Autodesk Fusion 360 part; units mm, degrees
(part 3 of 4)
  line L277 (275.3106, 39.6541) -> (275.3106, 39.9415)
  line L278 (275.3106, 39.9415) -> (276.614, 39.9415)
  arc A250 (276.614, 39.9415) -> (277.114, 40.4415) centre (276.614, 40.4415) ccw
  line L279 (277.114, 40.4415) -> (277.114, 40.6099)
  arc A251 (277.614, 41.1099) -> (277.114, 40.6099) centre (277.614, 40.6099) ccw
  line L280 (277.614, 41.1099) -> (279.662, 41.1099)
  arc A252 (280.162, 40.6099) -> (279.662, 41.1099) centre (279.662, 40.6099) ccw
  line L281 (280.162, 40.6099) -> (280.162, 40.4415)
  arc A253 (280.162, 40.4415) -> (280.662, 39.9415) centre (280.662, 40.4415) ccw
  line L282 (280.662, 39.9415) -> (281.4654, 39.9415)
  arc A254 (281.9654, 39.4415) -> (281.4654, 39.9415) centre (281.4654, 39.4415) ccw
  line L283 (281.9654, 39.4415) -> (281.9654, 34.3455)
  arc A255 (281.9654, 34.3455) -> (282.4654, 33.8455) centre (282.4654, 34.3455) ccw
  arc A256 (212.075, 26.8375) -> (212.575, 26.3375) centre (212.575, 26.8375) ccw
  line L284 (212.075, 26.8375) -> (212.075, 39.8375)
  arc A257 (212.575, 40.3375) -> (212.075, 39.8375) centre (212.575, 39.8375) ccw
  line L285 (212.575, 40.3375) -> (225.575, 40.3375)
  arc A258 (226.075, 39.8375) -> (225.575, 40.3375) centre (225.575, 39.8375) ccw
  line L286 (226.075, 39.8375) -> (226.075, 26.8375)
  arc A259 (225.575, 26.3375) -> (226.075, 26.8375) centre (225.575, 26.8375) ccw
  line L287 (225.575, 26.3375) -> (212.575, 26.3375)
  arc A260 (83.4875, 83.9875) -> (83.9875, 83.4875) centre (83.9875, 83.9875) ccw
  line L288 (83.4875, 83.9875) -> (83.4875, 96.9875)
  arc A261 (83.9875, 97.4875) -> (83.4875, 96.9875) centre (83.9875, 96.9875) ccw
  line L289 (83.9875, 97.4875) -> (96.9875, 97.4875)
  arc A262 (97.4875, 96.9875) -> (96.9875, 97.4875) centre (96.9875, 96.9875) ccw
  line L290 (97.4875, 96.9875) -> (97.4875, 83.9875)
  arc A263 (96.9875, 83.4875) -> (97.4875, 83.9875) centre (96.9875, 83.9875) ccw
  line L291 (96.9875, 83.4875) -> (83.9875, 83.4875)
  arc A264 (193.025, 26.8375) -> (193.525, 26.3375) centre (193.525, 26.8375) ccw
  line L292 (193.025, 26.8375) -> (193.025, 39.8375)
  arc A265 (193.525, 40.3375) -> (193.025, 39.8375) centre (193.525, 39.8375) ccw
  line L293 (193.525, 40.3375) -> (206.525, 40.3375)
  arc A266 (207.025, 39.8375) -> (206.525, 40.3375) centre (206.525, 39.8375) ccw
  line L294 (207.025, 39.8375) -> (207.025, 26.8375)
  arc A267 (206.525, 26.3375) -> (207.025, 26.8375) centre (206.525, 26.8375) ccw
  line L295 (206.525, 26.3375) -> (193.525, 26.3375)
  arc A268 (159.6875, 3.025) -> (160.1875, 2.525) centre (160.1875, 3.025) ccw
  line L296 (159.6875, 3.025) -> (159.6875, 16.025)
  arc A269 (160.1875, 16.525) -> (159.6875, 16.025) centre (160.1875, 16.025) ccw
  line L297 (160.1875, 16.525) -> (173.1875, 16.525)
  arc A270 (173.6875, 16.025) -> (173.1875, 16.525) centre (173.1875, 16.025) ccw
  line L298 (173.6875, 16.025) -> (173.6875, 3.025)
  arc A271 (173.1875, 2.525) -> (173.6875, 3.025) centre (173.1875, 3.025) ccw
  line L299 (173.1875, 2.525) -> (160.1875, 2.525)
  arc A272 (269.225, 103.0375) -> (269.725, 102.5375) centre (269.725, 103.0375) ccw
  line L300 (269.225, 103.0375) -> (269.225, 116.0375)
  arc A273 (269.725, 116.5375) -> (269.225, 116.0375) centre (269.725, 116.0375) ccw
  line L301 (269.725, 116.5375) -> (282.725, 116.5375)
  arc A274 (283.225, 116.0375) -> (282.725, 116.5375) centre (282.725, 116.0375) ccw
  line L302 (283.225, 116.0375) -> (283.225, 103.0375)
  arc A275 (282.725, 102.5375) -> (283.225, 103.0375) centre (282.725, 103.0375) ccw
  line L303 (282.725, 102.5375) -> (269.725, 102.5375)
  arc A276 (288.275, 103.0375) -> (288.775, 102.5375) centre (288.775, 103.0375) ccw
  line L304 (288.275, 103.0375) -> (288.275, 116.0375)
  arc A277 (288.775, 116.5375) -> (288.275, 116.0375) centre (288.775, 116.0375) ccw
  line L305 (288.775, 116.5375) -> (301.775, 116.5375)
  arc A278 (302.275, 116.0375) -> (301.775, 116.5375) centre (301.775, 116.0375) ccw
  line L306 (302.275, 116.0375) -> (302.275, 103.0375)
  arc A279 (301.775, 102.5375) -> (302.275, 103.0375) centre (301.775, 103.0375) ccw
  line L307 (301.775, 102.5375) -> (288.775, 102.5375)
  arc A280 (140.6375, 3.025) -> (141.1375, 2.525) centre (141.1375, 3.025) ccw
  line L308 (140.6375, 3.025) -> (140.6375, 16.025)
  arc A281 (141.1375, 16.525) -> (140.6375, 16.025) centre (141.1375, 16.025) ccw
  line L309 (141.1375, 16.525) -> (154.1375, 16.525)
  arc A282 (154.6375, 16.025) -> (154.1375, 16.525) centre (154.1375, 16.025) ccw
  line L310 (154.6375, 16.025) -> (154.6375, 3.025)
  arc A283 (154.1375, 2.525) -> (154.6375, 3.025) centre (154.1375, 3.025) ccw
  line L311 (154.1375, 2.525) -> (141.1375, 2.525)
  arc A284 (288.275, 83.9875) -> (288.775, 83.4875) centre (288.775, 83.9875) ccw
  line L312 (288.275, 83.9875) -> (288.275, 96.9875)
  arc A285 (288.775, 97.4875) -> (288.275, 96.9875) centre (288.775, 96.9875) ccw
  line L313 (288.775, 97.4875) -> (301.775, 97.4875)
  arc A286 (302.275, 96.9875) -> (301.775, 97.4875) centre (301.775, 96.9875) ccw
  line L314 (302.275, 96.9875) -> (302.275, 83.9875)
  arc A287 (301.775, 83.4875) -> (302.275, 83.9875) centre (301.775, 83.9875) ccw
  line L315 (301.775, 83.4875) -> (288.775, 83.4875)
  arc A288 (35.8625, 3.025) -> (36.3625, 2.525) centre (36.3625, 3.025) ccw
  line L316 (35.8625, 3.025) -> (35.8625, 16.025)
  arc A289 (36.3625, 16.525) -> (35.8625, 16.025) centre (36.3625, 16.025) ccw
  line L317 (36.3625, 16.525) -> (49.3625, 16.525)
  arc A290 (49.8625, 16.025) -> (49.3625, 16.525) centre (49.3625, 16.025) ccw
  line L318 (49.8625, 16.025) -> (49.8625, 3.025)
  arc A291 (49.3625, 2.525) -> (49.8625, 3.025) centre (49.3625, 3.025) ccw
  line L319 (49.3625, 2.525) -> (36.3625, 2.525)
  arc A292 (231.125, 26.8375) -> (231.625, 26.3375) centre (231.625, 26.8375) ccw
  line L320 (231.125, 26.8375) -> (231.125, 39.8375)
  arc A293 (231.625, 40.3375) -> (231.125, 39.8375) centre (231.625, 39.8375) ccw
  line L321 (231.625, 40.3375) -> (244.625, 40.3375)
  arc A294 (245.125, 39.8375) -> (244.625, 40.3375) centre (244.625, 39.8375) ccw
  line L322 (245.125, 39.8375) -> (245.125, 26.8375)
  arc A295 (244.625, 26.3375) -> (245.125, 26.8375) centre (244.625, 26.8375) ccw
  line L323 (244.625, 26.3375) -> (231.625, 26.3375)
  arc A296 (183.5, 45.8875) -> (184, 45.3875) centre (184, 45.8875) ccw
  line L324 (183.5, 45.8875) -> (183.5, 58.8875)
  arc A297 (184, 59.3875) -> (183.5, 58.8875) centre (184, 58.8875) ccw
  line L325 (184, 59.3875) -> (197, 59.3875)
  arc A298 (197.5, 58.8875) -> (197, 59.3875) centre (197, 58.8875) ccw
  line L326 (197.5, 58.8875) -> (197.5, 45.8875)
  arc A299 (197, 45.3875) -> (197.5, 45.8875) centre (197, 45.8875) ccw
  line L327 (197, 45.3875) -> (184, 45.3875)
  arc A300 (93.0125, 64.9375) -> (93.5125, 64.4375) centre (93.5125, 64.9375) ccw
  line L328 (93.0125, 64.9375) -> (93.0125, 77.9375)
  arc A301 (93.5125, 78.4375) -> (93.0125, 77.9375) centre (93.5125, 77.9375) ccw
  line L329 (93.5125, 78.4375) -> (106.5125, 78.4375)
  arc A302 (107.0125, 77.9375) -> (106.5125, 78.4375) centre (106.5125, 77.9375) ccw
  line L330 (107.0125, 77.9375) -> (107.0125, 64.9375)
  arc A303 (106.5125, 64.4375) -> (107.0125, 64.9375) centre (106.5125, 64.9375) ccw
  line L331 (106.5125, 64.4375) -> (93.5125, 64.4375)
  arc A304 (164.45, 45.8875) -> (164.95, 45.3875) centre (164.95, 45.8875) ccw
  line L332 (164.45, 45.8875) -> (164.45, 58.8875)
  arc A305 (164.95, 59.3875) -> (164.45, 58.8875) centre (164.95, 58.8875) ccw
  line L333 (164.95, 59.3875) -> (177.95, 59.3875)
  arc A306 (178.45, 58.8875) -> (177.95, 59.3875) centre (177.95, 58.8875) ccw
  line L334 (178.45, 58.8875) -> (178.45, 45.8875)
  arc A307 (177.95, 45.3875) -> (178.45, 45.8875) centre (177.95, 45.8875) ccw
  line L335 (177.95, 45.3875) -> (164.95, 45.3875)
  arc A308 (9.6688, 64.9375) -> (10.1687, 64.4375) centre (10.1687, 64.9375) ccw
  line L336 (9.6688, 64.9375) -> (9.6687, 77.9375)
  arc A309 (10.1687, 78.4375) -> (9.6688, 77.9375) centre (10.1687, 77.9375) ccw
  line L337 (10.1687, 78.4375) -> (23.1687, 78.4375)
  arc A310 (23.6687, 77.9375) -> (23.1687, 78.4375) centre (23.1687, 77.9375) ccw
  line L338 (23.6687, 77.9375) -> (23.6687, 64.9375)
  arc A311 (23.1687, 64.4375) -> (23.6687, 64.9375) centre (23.1687, 64.9375) ccw
  line L339 (23.1687, 64.4375) -> (10.1687, 64.4375)
  arc A312 (240.65, 45.8875) -> (241.15, 45.3875) centre (241.15, 45.8875) ccw
  line L340 (240.65, 45.8875) -> (240.65, 58.8875)
  arc A313 (241.15, 59.3875) -> (240.65, 58.8875) centre (241.15, 58.8875) ccw
  line L341 (241.15, 59.3875) -> (254.15, 59.3875)
  arc A314 (254.65, 58.8875) -> (254.15, 59.3875) centre (254.15, 58.8875) ccw
  line L342 (254.65, 58.8875) -> (254.65, 45.8875)
  arc A315 (254.15, 45.3875) -> (254.65, 45.8875) centre (254.15, 45.8875) ccw
  line L343 (254.15, 45.3875) -> (241.15, 45.3875)
  arc A316 (54.9125, 64.9375) -> (55.4125, 64.4375) centre (55.4125, 64.9375) ccw
  line L344 (54.9125, 64.9375) -> (54.9125, 77.9375)
  arc A317 (55.4125, 78.4375) -> (54.9125, 77.9375) centre (55.4125, 77.9375) ccw
  line L345 (55.4125, 78.4375) -> (68.4125, 78.4375)
  arc A318 (68.9125, 77.9375) -> (68.4125, 78.4375) centre (68.4125, 77.9375) ccw
  line L346 (68.9125, 77.9375) -> (68.9125, 64.9375)
  arc A319 (68.4125, 64.4375) -> (68.9125, 64.9375) centre (68.4125, 64.9375) ccw
  line L347 (68.4125, 64.4375) -> (55.4125, 64.4375)
  arc A320 (112.0625, 64.9375) -> (112.5625, 64.4375) centre (112.5625, 64.9375) ccw
  line L348 (112.0625, 64.9375) -> (112.0625, 77.9375)
  arc A321 (112.5625, 78.4375) -> (112.0625, 77.9375) centre (112.5625, 77.9375) ccw
  line L349 (112.5625, 78.4375) -> (125.5625, 78.4375)
  arc A322 (126.0625, 77.9375) -> (125.5625, 78.4375) centre (125.5625, 77.9375) ccw
  line L350 (126.0625, 77.9375) -> (126.0625, 64.9375)
  arc A323 (125.5625, 64.4375) -> (126.0625, 64.9375) centre (125.5625, 64.9375) ccw
  line L351 (125.5625, 64.4375) -> (112.5625, 64.4375)
  line L352 (37.1966, 90.9955) -> (37.5603, 90.9955)
  line L353 (37.5603, 90.9955) -> (37.5603, 88.7015)
  arc A324 (37.0603, 88.2015) -> (37.5603, 88.7015) centre (37.0603, 88.7015) ccw
  line L354 (37.0603, 88.2015) -> (36.6967, 88.2015)
  line L355 (36.6967, 88.2015) -> (36.6967, 85.2979)
  arc A325 (36.1966, 84.7979) -> (36.6967, 85.2979) centre (36.1966, 85.2979) ccw
  line L356 (36.1966, 84.7979) -> (30.5419, 84.7979)
  arc A326 (30.0418, 85.2979) -> (30.5419, 84.7979) centre (30.5419, 85.2979) ccw
  line L357 (30.0418, 85.2979) -> (30.0419, 85.6107)
  line L358 (30.0419, 85.6107) -> (28.4312, 85.6107)
  line L359 (28.4313, 85.6107) -> (28.4313, 83.9875)
  arc A327 (27.9312, 83.4875) -> (28.4313, 83.9875) centre (27.9312, 83.9875) ccw
  line L360 (27.9312, 83.4875) -> (14.9313, 83.4875)
  arc A328 (14.4313, 83.9875) -> (14.9313, 83.4875) centre (14.9313, 83.9875) ccw
  line L361 (14.4313, 83.9875) -> (14.4313, 85.6107)
  line L362 (14.4313, 85.6107) -> (12.8207, 85.6107)
  line L363 (12.8207, 85.6107) -> (12.8207, 85.2979)
  arc A329 (12.3207, 84.7979) -> (12.8207, 85.2979) centre (12.3207, 85.2979) ccw
  line L364 (12.3207, 84.7979) -> (6.6659, 84.7979)
  arc A330 (6.1658, 85.2979) -> (6.6658, 84.7979) centre (6.6658, 85.2979) ccw
  line L365 (6.1658, 85.2979) -> (6.1659, 88.2015)
  line L366 (6.1659, 88.2015) -> (5.8022, 88.2015)
  arc A331 (5.3022, 88.7015) -> (5.8022, 88.2015) centre (5.8022, 88.7015) ccw
  line L367 (5.3022, 88.7015) -> (5.3023, 90.9955)
  line L368 (5.3023, 90.9955) -> (5.6659, 90.9955)
  arc A332 (5.6658, 90.9955) -> (6.1658, 91.4955) centre (5.6658, 91.4955) ccw
  line L369 (6.1658, 91.4955) -> (6.1659, 96.5915)
  arc A333 (6.6658, 97.0915) -> (6.1658, 96.5915) centre (6.6658, 96.5915) ccw
  line L370 (6.6658, 97.0915) -> (7.4693, 97.0915)
  arc A334 (7.4693, 97.0915) -> (7.9693, 97.5915) centre (7.4692, 97.5915) ccw
  line L371 (7.9693, 97.5915) -> (7.9692, 97.7599)
  arc A335 (8.4693, 98.2599) -> (7.9692, 97.7599) centre (8.4693, 97.7599) ccw
  line L372 (8.4693, 98.2599) -> (10.5173, 98.2599)
  arc A336 (11.0173, 97.7599) -> (10.5173, 98.2599) centre (10.5173, 97.7599) ccw
  line L373 (11.0173, 97.7599) -> (11.0173, 97.5915)
  arc A337 (11.0173, 97.5915) -> (11.5173, 97.0915) centre (11.5172, 97.5915) ccw
  line L374 (11.5173, 97.0915) -> (12.8207, 97.0915)
  line L375 (12.8207, 97.0915) -> (12.8206, 96.8041)
  arc A338 (12.8206, 96.8041) -> (13.3207, 96.3041) centre (13.3206, 96.8041) ccw
  line L376 (13.3207, 96.3041) -> (14.4313, 96.3041)
  line L377 (14.4313, 96.3041) -> (14.4313, 96.9875)
  arc A339 (14.9313, 97.4875) -> (14.4312, 96.9875) centre (14.9313, 96.9875) ccw
  line L378 (14.9313, 97.4875) -> (27.9312, 97.4875)
  arc A340 (28.4313, 96.9875) -> (27.9312, 97.4875) centre (27.9312, 96.9875) ccw
  line L379 (28.4313, 96.9875) -> (28.4313, 96.3041)
  line L380 (28.4313, 96.3041) -> (29.5419, 96.3041)
  arc A341 (29.5419, 96.3041) -> (30.0418, 96.8041) centre (29.5419, 96.8041) ccw
  line L381 (30.0418, 96.8041) -> (30.0419, 97.0915)
  line L382 (30.0419, 97.0915) -> (31.3452, 97.0915)
  arc A342 (31.3452, 97.0915) -> (31.8453, 97.5915) centre (31.3452, 97.5915) ccw
  line L383 (31.8453, 97.5915) -> (31.8453, 97.7599)
  arc A343 (32.3453, 98.2599) -> (31.8452, 97.7599) centre (32.3453, 97.7599) ccw
  line L384 (32.3453, 98.2599) -> (34.3933, 98.2599)
  arc A344 (34.8933, 97.7599) -> (34.3933, 98.2599) centre (34.3933, 97.7599) ccw
  line L385 (34.8933, 97.7599) -> (34.8933, 97.5915)
  arc A345 (34.8933, 97.5915) -> (35.3933, 97.0915) centre (35.3932, 97.5915) ccw
  line L386 (35.3933, 97.0915) -> (36.1966, 97.0915)
  arc A346 (36.6967, 96.5915) -> (36.1966, 97.0915) centre (36.1966, 96.5915) ccw
  line L387 (36.6967, 96.5915) -> (36.6966, 91.4955)
  arc A347 (36.6966, 91.4955) -> (37.1966, 90.9955) centre (37.1967, 91.4955) ccw
  arc A348 (64.4375, 83.9875) -> (64.9375, 83.4875) centre (64.9375, 83.9875) ccw
  line L388 (64.4375, 83.9875) -> (64.4375, 96.9875)
  arc A349 (64.9375, 97.4875) -> (64.4375, 96.9875) centre (64.9375, 96.9875) ccw
  line L389 (64.9375, 97.4875) -> (77.9375, 97.4875)
  arc A350 (78.4375, 96.9875) -> (77.9375, 97.4875) centre (77.9375, 96.9875) ccw
  line L390 (78.4375, 96.9875) -> (78.4375, 83.9875)
  arc A351 (77.9375, 83.4875) -> (78.4375, 83.9875) centre (77.9375, 83.9875) ccw
  line L391 (77.9375, 83.4875) -> (64.9375, 83.4875)
  arc A352 (93.0125, 3.025) -> (93.5125, 2.525) centre (93.5125, 3.025) ccw
  line L392 (93.0125, 3.025) -> (93.0125, 16.025)
  arc A353 (93.5125, 16.525) -> (93.0125, 16.025) centre (93.5125, 16.025) ccw
  line L393 (93.5125, 16.525) -> (106.5125, 16.525)
  arc A354 (107.0125, 16.025) -> (106.5125, 16.525) centre (106.5125, 16.025) ccw
  line L394 (107.0125, 16.025) -> (107.0125, 3.025)
  arc A355 (106.5125, 2.525) -> (107.0125, 3.025) centre (106.5125, 3.025) ccw
  line L395 (106.5125, 2.525) -> (93.5125, 2.525)
  arc A356 (197.7875, 83.9875) -> (198.2875, 83.4875) centre (198.2875, 83.9875) ccw
  line L396 (197.7875, 83.9875) -> (197.7875, 96.9875)
  arc A357 (198.2875, 97.4875) -> (197.7875, 96.9875) centre (198.2875, 96.9875) ccw
  line L397 (198.2875, 97.4875) -> (211.2875, 97.4875)
  arc A358 (211.7875, 96.9875) -> (211.2875, 97.4875) centre (211.2875, 96.9875) ccw
  line L398 (211.7875, 96.9875) -> (211.7875, 83.9875)
  arc A359 (211.2875, 83.4875) -> (211.7875, 83.9875) centre (211.2875, 83.9875) ccw
  line L399 (211.2875, 83.4875) -> (198.2875, 83.4875)
  line L400 (280.0842, 71.9455) -> (280.4477, 71.9455)
  line L401 (280.4478, 71.9455) -> (280.4478, 69.6515)
  arc A360 (279.9477, 69.1515) -> (280.4477, 69.6515) centre (279.9477, 69.6515) ccw
  line L402 (279.9477, 69.1515) -> (279.5842, 69.1515)
  line L403 (279.5842, 69.1515) -> (279.5842, 66.2479)
  arc A361 (279.0842, 65.7479) -> (279.5842, 66.2479) centre (279.0842, 66.2479) ccw
  line L404 (279.0842, 65.7479) -> (273.4293, 65.7479)
  arc A362 (272.9293, 66.2479) -> (273.4293, 65.7479) centre (273.4293, 66.2479) ccw
  line L405 (272.9293, 66.2479) -> (272.9293, 66.5607)
  line L406 (272.9293, 66.5607) -> (271.3188, 66.5607)
  line L407 (271.3188, 66.5607) -> (271.3188, 64.9375)
  arc A363 (270.8188, 64.4375) -> (271.3188, 64.9375) centre (270.8188, 64.9375) ccw
  line L408 (270.8188, 64.4375) -> (257.8188, 64.4375)
  arc A364 (257.3188, 64.9375) -> (257.8188, 64.4375) centre (257.8188, 64.9375) ccw
  line L409 (257.3188, 64.9375) -> (257.3188, 66.5607)
  line L410 (257.3188, 66.5607) -> (255.7081, 66.5607)
  line L411 (255.7081, 66.5607) -> (255.7081, 66.2479)
  arc A365 (255.2081, 65.7479) -> (255.7081, 66.2479) centre (255.2081, 66.2479) ccw
  line L412 (255.2081, 65.7479) -> (249.5534, 65.7479)
  arc A366 (249.0534, 66.2479) -> (249.5534, 65.7479) centre (249.5534, 66.2479) ccw
  line L413 (249.0534, 66.2479) -> (249.0534, 69.1515)
  line L414 (249.0534, 69.1515) -> (248.6898, 69.1515)
  arc A367 (248.1898, 69.6515) -> (248.6898, 69.1515) centre (248.6898, 69.6515) ccw
  line L415 (248.1898, 69.6515) -> (248.1898, 71.9455)
  line L416 (248.1898, 71.9455) -> (248.5533, 71.9455)
  arc A368 (248.5533, 71.9455) -> (249.0533, 72.4455) centre (248.5534, 72.4455) ccw
  line L417 (249.0534, 72.4455) -> (249.0534, 77.5415)
  arc A369 (249.5534, 78.0415) -> (249.0534, 77.5415) centre (249.5534, 77.5415) ccw
  line L418 (249.5534, 78.0415) -> (250.3568, 78.0415)
  arc A370 (250.3568, 78.0415) -> (250.8568, 78.5415) centre (250.3568, 78.5415) ccw
  line L419 (250.8568, 78.5415) -> (250.8568, 78.7099)
  arc A371 (251.3568, 79.2099) -> (250.8568, 78.7099) centre (251.3568, 78.7099) ccw
  line L420 (251.3568, 79.2099) -> (253.4048, 79.2099)
  arc A372 (253.9048, 78.7099) -> (253.4048, 79.2099) centre (253.4048, 78.7099) ccw
  line L421 (253.9048, 78.7099) -> (253.9048, 78.5415)
  arc A373 (253.9048, 78.5415) -> (254.4048, 78.0415) centre (254.4047, 78.5415) ccw
  line L422 (254.4048, 78.0415) -> (255.7081, 78.0415)
  line L423 (255.7081, 78.0415) -> (255.7081, 77.7541)
  arc A374 (255.7081, 77.7541) -> (256.2081, 77.2541) centre (256.2082, 77.7541) ccw
  line L424 (256.2081, 77.2541) -> (257.3188, 77.2541)
  line L425 (257.3188, 77.2541) -> (257.3188, 77.9375)
  arc A375 (257.8188, 78.4375) -> (257.3188, 77.9375) centre (257.8188, 77.9375) ccw
  line L426 (257.8188, 78.4375) -> (270.8188, 78.4375)
  arc A376 (271.3188, 77.9375) -> (270.8188, 78.4375) centre (270.8188, 77.9375) ccw
  line L427 (271.3188, 77.9375) -> (271.3188, 77.2541)
  line L428 (271.3188, 77.2541) -> (272.4293, 77.2541)
  arc A377 (272.4293, 77.2541) -> (272.9293, 77.7541) centre (272.4293, 77.7541) ccw
  line L429 (272.9293, 77.7541) -> (272.9293, 78.0415)
  line L430 (272.9293, 78.0415) -> (274.2328, 78.0415)
  arc A378 (274.2328, 78.0415) -> (274.7327, 78.5415) centre (274.2328, 78.5415) ccw
  line L431 (274.7328, 78.5415) -> (274.7328, 78.7099)
  arc A379 (275.2328, 79.2099) -> (274.7328, 78.7099) centre (275.2328, 78.7099) ccw
  line L432 (275.2328, 79.2099) -> (277.2808, 79.2099)
  arc A380 (277.7808, 78.7099) -> (277.2808, 79.2099) centre (277.2808, 78.7099) ccw
  line L433 (277.7808, 78.7099) -> (277.7808, 78.5415)
  arc A381 (277.7808, 78.5415) -> (278.2808, 78.0415) centre (278.2808, 78.5415) ccw
  line L434 (278.2808, 78.0415) -> (279.0842, 78.0415)
  arc A382 (279.5842, 77.5415) -> (279.0842, 78.0415) centre (279.0842, 77.5415) ccw
  line L435 (279.5842, 77.5415) -> (279.5842, 72.4455)
  arc A383 (279.5842, 72.4455) -> (280.0842, 71.9455) centre (280.0842, 72.4455) ccw
  arc A384 (2.525, 3.025) -> (3.025, 2.525) centre (3.025, 3.025) ccw
  line L436 (2.525, 3.025) -> (2.525, 16.025)
  arc A385 (3.025, 16.525) -> (2.525, 16.025) centre (3.025, 16.025) ccw
  line L437 (3.025, 16.525) -> (16.025, 16.525)
  arc A386 (16.525, 16.025) -> (16.025, 16.525) centre (16.025, 16.025) ccw
  line L438 (16.525, 16.025) -> (16.525, 3.025)
  arc A387 (16.025, 2.525) -> (16.525, 3.025) centre (16.025, 3.025) ccw
  line L439 (16.025, 2.525) -> (3.025, 2.525)
  arc A388 (140.6375, 83.9875) -> (141.1375, 83.4875) centre (141.1375, 83.9875) ccw
  line L440 (140.6375, 83.9875) -> (140.6375, 96.9875)
  arc A389 (141.1375, 97.4875) -> (140.6375, 96.9875) centre (141.1375, 96.9875) ccw
  line L441 (141.1375, 97.4875) -> (154.1375, 97.4875)
  arc A390 (154.6375, 96.9875) -> (154.1375, 97.4875) centre (154.1375, 96.9875) ccw
  line L442 (154.6375, 96.9875) -> (154.6375, 83.9875)
  arc A391 (154.1375, 83.4875) -> (154.6375, 83.9875) centre (154.1375, 83.9875) ccw
  line L443 (154.1375, 83.4875) -> (141.1375, 83.4875)
  arc A392 (178.7375, 83.9875) -> (179.2375, 83.4875) centre (179.2375, 83.9875) ccw
  line L444 (178.7375, 83.9875) -> (178.7375, 96.9875)
  arc A393 (179.2375, 97.4875) -> (178.7375, 96.9875) centre (179.2375, 96.9875) ccw
  line L445 (179.2375, 97.4875) -> (192.2375, 97.4875)
  arc A394 (192.7375, 96.9875) -> (192.2375, 97.4875) centre (192.2375, 96.9875) ccw
  line L446 (192.7375, 96.9875) -> (192.7375, 83.9875)
  arc A395 (192.2375, 83.4875) -> (192.7375, 83.9875) centre (192.2375, 83.9875) ccw
  line L447 (192.2375, 83.4875) -> (179.2375, 83.4875)
  arc A396 (173.975, 26.8375) -> (174.475, 26.3375) centre (174.475, 26.8375) ccw
  line L448 (173.975, 26.8375) -> (173.975, 39.8375)
  arc A397 (174.475, 40.3375) -> (173.975, 39.8375) centre (174.475, 39.8375) ccw
  line L449 (174.475, 40.3375) -> (187.475, 40.3375)
  arc A398 (187.975, 39.8375) -> (187.475, 40.3375) centre (187.475, 39.8375) ccw
  line L450 (187.975, 39.8375) -> (187.975, 26.8375)
  arc A399 (187.475, 26.3375) -> (187.975, 26.8375) centre (187.475, 26.8375) ccw
  line L451 (187.475, 26.3375) -> (174.475, 26.3375)
  arc A400 (131.1125, 64.9375) -> (131.6125, 64.4375) centre (131.6125, 64.9375) ccw
  line L452 (131.1125, 64.9375) -> (131.1125, 77.9375)
  arc A401 (131.6125, 78.4375) -> (131.1125, 77.9375) centre (131.6125, 77.9375) ccw
  line L453 (131.6125, 78.4375) -> (144.6125, 78.4375)
  arc A402 (145.1125, 77.9375) -> (144.6125, 78.4375) centre (144.6125, 77.9375) ccw
  line L454 (145.1125, 77.9375) -> (145.1125, 64.9375)
  arc A403 (144.6125, 64.4375) -> (145.1125, 64.9375) centre (144.6125, 64.9375) ccw
  line L455 (144.6125, 64.4375) -> (131.6125, 64.4375)
  arc A404 (150.1625, 64.9375) -> (150.6625, 64.4375) centre (150.6625, 64.9375) ccw
  line L456 (150.1625, 64.9375) -> (150.1625, 77.9375)
  arc A405 (150.6625, 78.4375) -> (150.1625, 77.9375) centre (150.6625, 77.9375) ccw
  line L457 (150.6625, 78.4375) -> (163.6625, 78.4375)
  arc A406 (164.1625, 77.9375) -> (163.6625, 78.4375) centre (163.6625, 77.9375) ccw
  line L458 (164.1625, 77.9375) -> (164.1625, 64.9375)
  arc A407 (163.6625, 64.4375) -> (164.1625, 64.9375) centre (163.6625, 64.9375) ccw
  line L459 (163.6625, 64.4375) -> (150.6625, 64.4375)
  arc A408 (202.55, 45.8875) -> (203.05, 45.3875) centre (203.05, 45.8875) ccw
  line L460 (202.55, 45.8875) -> (202.55, 58.8875)
  arc A409 (203.05, 59.3875) -> (202.55, 58.8875) centre (203.05, 58.8875) ccw
  line L461 (203.05, 59.3875) -> (216.05, 59.3875)
  arc A410 (216.55, 58.8875) -> (216.05, 59.3875) centre (216.05, 58.8875) ccw
  line L462 (216.55, 58.8875) -> (216.55, 45.8875)
  arc A411 (216.05, 45.3875) -> (216.55, 45.8875) centre (216.05, 45.8875) ccw
  line L463 (216.05, 45.3875) -> (203.05, 45.3875)
  arc A412 (88.25, 45.8875) -> (88.75, 45.3875) centre (88.75, 45.8875) ccw
  line L464 (88.25, 45.8875) -> (88.25, 58.8875)
  arc A413 (88.75, 59.3875) -> (88.25, 58.8875) centre (88.75, 58.8875) ccw
  line L465 (88.75, 59.3875) -> (101.75, 59.3875)
  arc A414 (102.25, 58.8875) -> (101.75, 59.3875) centre (101.75, 58.8875) ccw
  line L466 (102.25, 58.8875) -> (102.25, 45.8875)
  arc A415 (101.75, 45.3875) -> (102.25, 45.8875) centre (101.75, 45.8875) ccw
  line L467 (101.75, 45.3875) -> (88.75, 45.3875)
  arc A416 (97.775, 26.8375) -> (98.275, 26.3375) centre (98.275, 26.8375) ccw
  line L468 (97.775, 26.8375) -> (97.775, 39.8375)
  arc A417 (98.275, 40.3375) -> (97.775, 39.8375) centre (98.275, 39.8375) ccw
  line L469 (98.275, 40.3375) -> (111.275, 40.3375)
  arc A418 (111.775, 39.8375) -> (111.275, 40.3375) centre (111.275, 39.8375) ccw
  line L470 (111.775, 39.8375) -> (111.775, 26.8375)
  arc A419 (111.275, 26.3375) -> (111.775, 26.8375) centre (111.275, 26.8375) ccw
  line L471 (111.275, 26.3375) -> (98.275, 26.3375)
  line L472 (157, 21) -> (157, -10)
  line L473 (157, 21) -> (152.4, 21)
  line L474 (152.4, 21) -> (152.4, 43)
  line L475 (152.4, 43) -> (162, 43)
  line L476 (162, 43) -> (162, 62)
  line L477 (162, 62) -> (147.5, 62)
  line L478 (147.5, 62) -> (147.5, 81)
  line L479 (147.5, 81) -> (157, 81)
  line L480 (157, 81) -> (157, 130.1996)
  dimension "d39" = 14.5
  constraint coincident L214 L472.end
  constraint perpendicular L214 L472
  constraint perpendicular L472 L473
  constraint perpendicular L83 L474
  constraint perpendicular L472 L475
  constraint perpendicular L83 L476
  constraint perpendicular L476 L477
  constraint perpendicular L477 L478
  constraint perpendicular L476 L479
  constraint coincident L224 L480.end
  constraint perpendicular L224 L480
  measures "d39" distance of L476.end L477.end
split "Split1" by curves path "Sketch2" along L480 L479 L478 L477 L476 L475 L474 L473 L472 bodies 1 makes body 2 at (131.2104, -125.6456, 0)
sketch "Sketch3" plane through (0, 0, 0) normal (0, 0, -1) x (1, 0, 0)
  line L0 (157, 81) -> (157, 107.2375)
  line L1 (157, 107.2375) -> (142.7312, 107.2375)
  line L2 (142.7312, 107.2375) -> (142.7312, 103.0375)
  arc A0 (142.2312, 102.5375) -> (142.7312, 103.0375) centre (142.2312, 103.0375) ccw
  line L3 (142.2312, 102.5375) -> (129.2312, 102.5375)
  arc A1 (128.7312, 103.0375) -> (129.2312, 102.5375) centre (129.2312, 103.0375) ccw
  line L4 (128.7312, 103.0375) -> (128.7313, 107.2375)
  line L5 (128.7312, 107.2375) -> (89.5587, 107.2375)
  arc A2 (89.5587, 107.2375) -> (89.0587, 106.7375) centre (89.5587, 106.7375) ccw
  line L6 (89.0587, 106.7375) -> (89.0587, 104.3479)
  arc A3 (88.5587, 103.8479) -> (89.0587, 104.3479) centre (88.5587, 104.3479) ccw
  line L7 (88.5587, 103.8479) -> (82.9039, 103.8479)
  arc A4 (82.4039, 104.3479) -> (82.9039, 103.8479) centre (82.9039, 104.3479) ccw
  line L8 (82.4039, 104.3479) -> (82.4039, 107.2515)
  line L9 (82.4039, 107.2515) -> (82.0403, 107.2515)
  arc A5 (81.5402, 107.7515) -> (82.0403, 107.2515) centre (82.0403, 107.7515) ccw
  line L10 (81.5402, 107.7515) -> (81.5403, 110.0455)
  line L11 (81.5403, 110.0455) -> (81.9039, 110.0455)
  arc A6 (81.9039, 110.0455) -> (82.4039, 110.5455) centre (81.9038, 110.5455) ccw
  line L12 (82.4039, 110.5455) -> (82.4039, 115.6415)
  arc A7 (82.9039, 116.1415) -> (82.4039, 115.6415) centre (82.9039, 115.6415) ccw
  line L13 (82.9039, 116.1415) -> (83.7073, 116.1415)
  arc A8 (83.7073, 116.1415) -> (84.2073, 116.6415) centre (83.7073, 116.6415) ccw
  line L14 (84.2073, 116.6415) -> (84.2073, 116.8099)
  arc A9 (84.7073, 117.3099) -> (84.2073, 116.8099) centre (84.7073, 116.8099) ccw
  line L15 (84.7073, 117.3099) -> (86.7553, 117.3099)
  arc A10 (87.2552, 116.8099) -> (86.7553, 117.3099) centre (86.7553, 116.8099) ccw
  line L16 (87.2552, 116.8099) -> (87.2553, 116.6415)
  arc A11 (87.2553, 116.6415) -> (87.7553, 116.1415) centre (87.7552, 116.6415) ccw
  line L17 (87.7553, 116.1415) -> (88.5587, 116.1415)
  arc A12 (89.0587, 115.6415) -> (88.5587, 116.1415) centre (88.5587, 115.6415) ccw
  line L18 (89.0587, 115.6415) -> (89.0587, 112.3375)
  arc A13 (89.0587, 112.3375) -> (89.5587, 111.8375) centre (89.5587, 112.3375) ccw
  line L19 (89.5587, 111.8375) -> (128.7312, 111.8375)
  line L20 (128.7312, 111.8375) -> (128.7312, 116.0375)
  arc A14 (129.2312, 116.5375) -> (128.7312, 116.0375) centre (129.2312, 116.0375) ccw
  line L21 (129.2312, 116.5375) -> (142.2312, 116.5375)
  arc A15 (142.7312, 116.0375) -> (142.2312, 116.5375) centre (142.2312, 116.0375) ccw
  line L22 (142.7312, 116.0375) -> (142.7312, 111.8375)
  line L23 (142.7312, 111.8375) -> (157, 111.8375)
  line L24 (157, 111.8375) -> (157, 130.1996)
  line L25 (157, 130.1996) -> (107.4, 130.1996)
  arc A16 (107.4, 130.1996) -> (102.4, 125.1996) centre (107.4, 125.1996) ccw
  line L26 (102.4, 125.1996) -> (102.4, 123.1996)
  line L27 (102.4, 123.1996) -> (31, 123.1996)
  line L28 (31, 123.1996) -> (31, 125.1996)
  arc A17 (31, 125.1996) -> (26, 130.1996) centre (26, 125.1996) ccw
  line L29 (26, 130.1996) -> (1, 130.1996)
  arc A18 (1, 130.1996) -> (-4, 125.1996) centre (1, 125.1996) ccw
  line L30 (-4, 125.1996) -> (-4, -5)
  arc A19 (-4, -5) -> (1, -10) centre (1, -5) ccw
  line L31 (1, -10) -> (26, -10)
  arc A20 (26, -10) -> (31, -5) centre (26, -5) ccw
  line L32 (31, -5) -> (31, -3)
  line L33 (31, -3) -> (102.4, -3)
  line L34 (102.4, -3) -> (102.4, -5)
  arc A21 (102.4, -5) -> (107.4, -10) centre (107.4, -5) ccw
  line L35 (107.4, -10) -> (157, -10)
  line L36 (157, -10) -> (157, 21)
  line L37 (157, 21) -> (152.4, 21)
  line L38 (152.4, 21) -> (152.4, 43)
  line L39 (152.4, 43) -> (162, 43)
  line L40 (162, 43) -> (162, 62)
  line L41 (162, 62) -> (147.5, 62)
  line L42 (147.5, 62) -> (147.5, 81)
  line L43 (147.5, 81) -> (157, 81)
  arc A22 (97.775, 26.8375) -> (98.275, 26.3375) centre (98.275, 26.8375) ccw
  line L44 (97.775, 26.8375) -> (97.775, 39.8375)
  arc A23 (98.275, 40.3375) -> (97.775, 39.8375) centre (98.275, 39.8375) ccw
  line L45 (98.275, 40.3375) -> (111.275, 40.3375)
  arc A24 (111.775, 39.8375) -> (111.275, 40.3375) centre (111.275, 39.8375) ccw
  line L46 (111.775, 39.8375) -> (111.775, 26.8375)
  arc A25 (111.275, 26.3375) -> (111.775, 26.8375) centre (111.275, 26.8375) ccw
  line L47 (111.275, 26.3375) -> (98.275, 26.3375)
  arc A26 (69.2, 45.8875) -> (69.7, 45.3875) centre (69.7, 45.8875) ccw
  line L48 (69.2, 45.8875) -> (69.2, 58.8875)
  arc A27 (69.7, 59.3875) -> (69.2, 58.8875) centre (69.7, 58.8875) ccw
  line L49 (69.7, 59.3875) -> (82.7, 59.3875)
  arc A28 (83.2, 58.8875) -> (82.7, 59.3875) centre (82.7, 58.8875) ccw
  line L50 (83.2, 58.8875) -> (83.2, 45.8875)
  arc A29 (82.7, 45.3875) -> (83.2, 45.8875) centre (82.7, 45.8875) ccw
  line L51 (82.7, 45.3875) -> (69.7, 45.3875)
  arc A30 (140.6375, 83.9875) -> (141.1375, 83.4875) centre (141.1375, 83.9875) ccw
  line L52 (140.6375, 83.9875) -> (140.6375, 96.9875)
  arc A31 (141.1375, 97.4875) -> (140.6375, 96.9875) centre (141.1375, 96.9875) ccw
  line L53 (141.1375, 97.4875) -> (154.1375, 97.4875)
  arc A32 (154.6375, 96.9875) -> (154.1375, 97.4875) centre (154.1375, 96.9875) ccw
  line L54 (154.6375, 96.9875) -> (154.6375, 83.9875)
  arc A33 (154.1375, 83.4875) -> (154.6375, 83.9875) centre (154.1375, 83.9875) ccw
  line L55 (154.1375, 83.4875) -> (141.1375, 83.4875)
  arc A34 (50.15, 45.8875) -> (50.65, 45.3875) centre (50.65, 45.8875) ccw
  line L56 (50.15, 45.8875) -> (50.15, 58.8875)
  arc A35 (50.65, 59.3875) -> (50.15, 58.8875) centre (50.65, 58.8875) ccw
  line L57 (50.65, 59.3875) -> (63.65, 59.3875)
  arc A36 (64.15, 58.8875) -> (63.65, 59.3875) centre (63.65, 58.8875) ccw
  line L58 (64.15, 58.8875) -> (64.15, 45.8875)
  arc A37 (63.65, 45.3875) -> (64.15, 45.8875) centre (63.65, 45.8875) ccw
  line L59 (63.65, 45.3875) -> (50.65, 45.3875)
  arc A38 (9.6688, 64.9375) -> (10.1687, 64.4375) centre (10.1687, 64.9375) ccw
  line L60 (9.6688, 64.9375) -> (9.6687, 77.9375)
  arc A39 (10.1687, 78.4375) -> (9.6688, 77.9375) centre (10.1687, 77.9375) ccw
  line L61 (10.1687, 78.4375) -> (23.1687, 78.4375)
  arc A40 (23.6687, 77.9375) -> (23.1687, 78.4375) centre (23.1687, 77.9375) ccw
  line L62 (23.6687, 77.9375) -> (23.6687, 64.9375)
  arc A41 (23.1687, 64.4375) -> (23.6687, 64.9375) centre (23.1687, 64.9375) ccw
  line L63 (23.1687, 64.4375) -> (10.1687, 64.4375)
  arc A42 (102.5375, 83.9875) -> (103.0375, 83.4875) centre (103.0375, 83.9875) ccw
  line L64 (102.5375, 83.9875) -> (102.5375, 96.9875)
  arc A43 (103.0375, 97.4875) -> (102.5375, 96.9875) centre (103.0375, 96.9875) ccw
  line L65 (103.0375, 97.4875) -> (116.0375, 97.4875)
  arc A44 (116.5375, 96.9875) -> (116.0375, 97.4875) centre (116.0375, 96.9875) ccw
  line L66 (116.5375, 96.9875) -> (116.5375, 83.9875)
  arc A45 (116.0375, 83.4875) -> (116.5375, 83.9875) centre (116.0375, 83.9875) ccw
  line L67 (116.0375, 83.4875) -> (103.0375, 83.4875)
  arc A46 (121.5875, 83.9875) -> (122.0875, 83.4875) centre (122.0875, 83.9875) ccw
  line L68 (121.5875, 83.9875) -> (121.5875, 96.9875)
  arc A47 (122.0875, 97.4875) -> (121.5875, 96.9875) centre (122.0875, 96.9875) ccw
  line L69 (122.0875, 97.4875) -> (135.0875, 97.4875)
  arc A48 (135.5875, 96.9875) -> (135.0875, 97.4875) centre (135.0875, 96.9875) ccw
  line L70 (135.5875, 96.9875) -> (135.5875, 83.9875)
  arc A49 (135.0875, 83.4875) -> (135.5875, 83.9875) centre (135.0875, 83.9875) ccw
  line L71 (135.0875, 83.4875) -> (122.0875, 83.4875)
  arc A50 (112.0625, 64.9375) -> (112.5625, 64.4375) centre (112.5625, 64.9375) ccw
  line L72 (112.0625, 64.9375) -> (112.0625, 77.9375)
  arc A51 (112.5625, 78.4375) -> (112.0625, 77.9375) centre (112.5625, 77.9375) ccw
  line L73 (112.5625, 78.4375) -> (125.5625, 78.4375)
  arc A52 (126.0625, 77.9375) -> (125.5625, 78.4375) centre (125.5625, 77.9375) ccw
  line L74 (126.0625, 77.9375) -> (126.0625, 64.9375)
  arc A53 (125.5625, 64.4375) -> (126.0625, 64.9375) centre (125.5625, 64.9375) ccw
  line L75 (125.5625, 64.4375) -> (112.5625, 64.4375)
  arc A54 (40.625, 26.8375) -> (41.125, 26.3375) centre (41.125, 26.8375) ccw
  line L76 (40.625, 26.8375) -> (40.625, 39.8375)
  arc A55 (41.125, 40.3375) -> (40.625, 39.8375) centre (41.125, 39.8375) ccw
  line L77 (41.125, 40.3375) -> (54.125, 40.3375)
  arc A56 (54.625, 39.8375) -> (54.125, 40.3375) centre (54.125, 39.8375) ccw
  line L78 (54.625, 39.8375) -> (54.625, 26.8375)
  arc A57 (54.125, 26.3375) -> (54.625, 26.8375) centre (54.125, 26.8375) ccw
  line L79 (54.125, 26.3375) -> (41.125, 26.3375)
  arc A58 (121.5875, 3.025) -> (122.0875, 2.525) centre (122.0875, 3.025) ccw
  line L80 (121.5875, 3.025) -> (121.5875, 16.025)
  arc A59 (122.0875, 16.525) -> (121.5875, 16.025) centre (122.0875, 16.025) ccw
  line L81 (122.0875, 16.525) -> (135.0875, 16.525)
  arc A60 (135.5875, 16.025) -> (135.0875, 16.525) centre (135.0875, 16.025) ccw
  line L82 (135.5875, 16.025) -> (135.5875, 3.025)
  arc A61 (135.0875, 2.525) -> (135.5875, 3.025) centre (135.0875, 3.025) ccw
  line L83 (135.0875, 2.525) -> (122.0875, 2.525)
  arc A62 (4.9062, 103.0375) -> (5.4062, 102.5375) centre (5.4062, 103.0375) ccw
  line L84 (4.9062, 103.0375) -> (4.9062, 116.0375)
  arc A63 (5.4062, 116.5375) -> (4.9062, 116.0375) centre (5.4062, 116.0375) ccw
  line L85 (5.4062, 116.5375) -> (18.4063, 116.5375)
  arc A64 (18.9063, 116.0375) -> (18.4062, 116.5375) centre (18.4062, 116.0375) ccw
  line L86 (18.9063, 116.0375) -> (18.9062, 103.0375)
  arc A65 (18.4062, 102.5375) -> (18.9063, 103.0375) centre (18.4062, 103.0375) ccw
  line L87 (18.4062, 102.5375) -> (5.4062, 102.5375)
  arc A66 (64.4375, 83.9875) -> (64.9375, 83.4875) centre (64.9375, 83.9875) ccw
  line L88 (64.4375, 83.9875) -> (64.4375, 96.9875)
  arc A67 (64.9375, 97.4875) -> (64.4375, 96.9875) centre (64.9375, 96.9875) ccw
  line L89 (64.9375, 97.4875) -> (77.9375, 97.4875)
  arc A68 (78.4375, 96.9875) -> (77.9375, 97.4875) centre (77.9375, 96.9875) ccw
  line L90 (78.4375, 96.9875) -> (78.4375, 83.9875)
  arc A69 (77.9375, 83.4875) -> (78.4375, 83.9875) centre (77.9375, 83.9875) ccw
  line L91 (77.9375, 83.4875) -> (64.9375, 83.4875)
  arc A70 (83.4875, 83.9875) -> (83.9875, 83.4875) centre (83.9875, 83.9875) ccw
  line L92 (83.4875, 83.9875) -> (83.4875, 96.9875)
  arc A71 (83.9875, 97.4875) -> (83.4875, 96.9875) centre (83.9875, 96.9875) ccw
  line L93 (83.9875, 97.4875) -> (96.9875, 97.4875)
  arc A72 (97.4875, 96.9875) -> (96.9875, 97.4875) centre (96.9875, 96.9875) ccw
  line L94 (97.4875, 96.9875) -> (97.4875, 83.9875)
  arc A73 (96.9875, 83.4875) -> (97.4875, 83.9875) centre (96.9875, 83.9875) ccw
  line L95 (96.9875, 83.4875) -> (83.9875, 83.4875)
  arc A74 (45.3875, 83.9875) -> (45.8875, 83.4875) centre (45.8875, 83.9875) ccw
  line L96 (45.3875, 83.9875) -> (45.3875, 96.9875)
  arc A75 (45.8875, 97.4875) -> (45.3875, 96.9875) centre (45.8875, 96.9875) ccw
  line L97 (45.8875, 97.4875) -> (58.8875, 97.4875)
  arc A76 (59.3875, 96.9875) -> (58.8875, 97.4875) centre (58.8875, 96.9875) ccw
  line L98 (59.3875, 96.9875) -> (59.3875, 83.9875)
  arc A77 (58.8875, 83.4875) -> (59.3875, 83.9875) centre (58.8875, 83.9875) ccw
  line L99 (58.8875, 83.4875) -> (45.8875, 83.4875)
  line L100 (37.1966, 90.9955) -> (37.5603, 90.9955)
  line L101 (37.5603, 90.9955) -> (37.5603, 88.7015)
  arc A78 (37.0603, 88.2015) -> (37.5603, 88.7015) centre (37.0603, 88.7015) ccw
  line L102 (37.0603, 88.2015) -> (36.6967, 88.2015)
  line L103 (36.6967, 88.2015) -> (36.6967, 85.2979)
  arc A79 (36.1966, 84.7979) -> (36.6967, 85.2979) centre (36.1966, 85.2979) ccw
  line L104 (36.1966, 84.7979) -> (30.5419, 84.7979)
  arc A80 (30.0418, 85.2979) -> (30.5419, 84.7979) centre (30.5419, 85.2979) ccw
  line L105 (30.0418, 85.2979) -> (30.0419, 85.6107)
  line L106 (30.0419, 85.6107) -> (28.4312, 85.6107)
  line L107 (28.4313, 85.6107) -> (28.4313, 83.9875)
  arc A81 (27.9312, 83.4875) -> (28.4313, 83.9875) centre (27.9312, 83.9875) ccw
  line L108 (27.9312, 83.4875) -> (14.9313, 83.4875)
  arc A82 (14.4313, 83.9875) -> (14.9313, 83.4875) centre (14.9313, 83.9875) ccw
  line L109 (14.4313, 83.9875) -> (14.4313, 85.6107)
  line L110 (14.4313, 85.6107) -> (12.8207, 85.6107)
  line L111 (12.8207, 85.6107) -> (12.8207, 85.2979)
  arc A83 (12.3207, 84.7979) -> (12.8207, 85.2979) centre (12.3207, 85.2979) ccw
  line L112 (12.3207, 84.7979) -> (6.6659, 84.7979)
  arc A84 (6.1658, 85.2979) -> (6.6658, 84.7979) centre (6.6658, 85.2979) ccw
  line L113 (6.1658, 85.2979) -> (6.1659, 88.2015)
  line L114 (6.1659, 88.2015) -> (5.8022, 88.2015)
  arc A85 (5.3022, 88.7015) -> (5.8022, 88.2015) centre (5.8022, 88.7015) ccw
  line L115 (5.3022, 88.7015) -> (5.3023, 90.9955)
  line L116 (5.3023, 90.9955) -> (5.6659, 90.9955)
  arc A86 (5.6658, 90.9955) -> (6.1658, 91.4955) centre (5.6658, 91.4955) ccw
  line L117 (6.1658, 91.4955) -> (6.1659, 96.5915)
  arc A87 (6.6658, 97.0915) -> (6.1658, 96.5915) centre (6.6658, 96.5915) ccw
  line L118 (6.6658, 97.0915) -> (7.4693, 97.0915)
  arc A88 (7.4693, 97.0915) -> (7.9693, 97.5915) centre (7.4692, 97.5915) ccw
  line L119 (7.9693, 97.5915) -> (7.9692, 97.7599)
  arc A89 (8.4693, 98.2599) -> (7.9692, 97.7599) centre (8.4693, 97.7599) ccw
  line L120 (8.4693, 98.2599) -> (10.5173, 98.2599)
  arc A90 (11.0173, 97.7599) -> (10.5173, 98.2599) centre (10.5173, 97.7599) ccw
  line L121 (11.0173, 97.7599) -> (11.0173, 97.5915)
  arc A91 (11.0173, 97.5915) -> (11.5173, 97.0915) centre (11.5172, 97.5915) ccw
  line L122 (11.5173, 97.0915) -> (12.8207, 97.0915)
  line L123 (12.8207, 97.0915) -> (12.8206, 96.8041)
  arc A92 (12.8206, 96.8041) -> (13.3207, 96.3041) centre (13.3206, 96.8041) ccw
  line L124 (13.3207, 96.3041) -> (14.4313, 96.3041)
  line L125 (14.4313, 96.3041) -> (14.4313, 96.9875)
  arc A93 (14.9313, 97.4875) -> (14.4312, 96.9875) centre (14.9313, 96.9875) ccw
  line L126 (14.9313, 97.4875) -> (27.9312, 97.4875)
  arc A94 (28.4313, 96.9875) -> (27.9312, 97.4875) centre (27.9312, 96.9875) ccw
  line L127 (28.4313, 96.9875) -> (28.4313, 96.3041)
  line L128 (28.4313, 96.3041) -> (29.5419, 96.3041)
  arc A95 (29.5419, 96.3041) -> (30.0418, 96.8041) centre (29.5419, 96.8041) ccw
  line L129 (30.0418, 96.8041) -> (30.0419, 97.0915)
  line L130 (30.0419, 97.0915) -> (31.3452, 97.0915)
  arc A96 (31.3452, 97.0915) -> (31.8453, 97.5915) centre (31.3452, 97.5915) ccw
  line L131 (31.8453, 97.5915) -> (31.8453, 97.7599)
  arc A97 (32.3453, 98.2599) -> (31.8452, 97.7599) centre (32.3453, 97.7599) ccw
  line L132 (32.3453, 98.2599) -> (34.3933, 98.2599)
  arc A98 (34.8933, 97.7599) -> (34.3933, 98.2599) centre (34.3933, 97.7599) ccw
  line L133 (34.8933, 97.7599) -> (34.8933, 97.5915)
  arc A99 (34.8933, 97.5915) -> (35.3933, 97.0915) centre (35.3932, 97.5915) ccw
  line L134 (35.3933, 97.0915) -> (36.1966, 97.0915)
  arc A100 (36.6967, 96.5915) -> (36.1966, 97.0915) centre (36.1966, 96.5915) ccw
  line L135 (36.6967, 96.5915) -> (36.6966, 91.4955)
  arc A101 (36.6966, 91.4955) -> (37.1966, 90.9955) centre (37.1967, 91.4955) ccw
  arc A102 (88.25, 45.8875) -> (88.75, 45.3875) centre (88.75, 45.8875) ccw
  line L136 (88.25, 45.8875) -> (88.25, 58.8875)
  arc A103 (88.75, 59.3875) -> (88.25, 58.8875) centre (88.75, 58.8875) ccw
  line L137 (88.75, 59.3875) -> (101.75, 59.3875)
  arc A104 (102.25, 58.8875) -> (101.75, 59.3875) centre (101.75, 58.8875) ccw
  line L138 (102.25, 58.8875) -> (102.25, 45.8875)
  arc A105 (101.75, 45.3875) -> (102.25, 45.8875) centre (101.75, 45.8875) ccw
  line L139 (101.75, 45.3875) -> (88.75, 45.3875)
  arc A106 (21.575, 26.8375) -> (22.075, 26.3375) centre (22.075, 26.8375) ccw
  line L140 (21.575, 26.8375) -> (21.575, 39.8375)
  arc A107 (22.075, 40.3375) -> (21.575, 39.8375) centre (22.075, 39.8375) ccw
  line L141 (22.075, 40.3375) -> (35.075, 40.3375)
  arc A108 (35.575, 39.8375) -> (35.075, 40.3375) centre (35.075, 39.8375) ccw
  line L142 (35.575, 39.8375) -> (35.575, 26.8375)
  arc A109 (35.075, 26.3375) -> (35.575, 26.8375) centre (35.075, 26.8375) ccw
  line L143 (35.075, 26.3375) -> (22.075, 26.3375)
  arc A110 (54.9125, 103.0375) -> (55.4125, 102.5375) centre (55.4125, 103.0375) ccw
  line L144 (54.9125, 103.0375) -> (54.9125, 116.0375)
  arc A111 (55.4125, 116.5375) -> (54.9125, 116.0375) centre (55.4125, 116.0375) ccw
  line L145 (55.4125, 116.5375) -> (68.4125, 116.5375)
  arc A112 (68.9125, 116.0375) -> (68.4125, 116.5375) centre (68.4125, 116.0375) ccw
  line L146 (68.9125, 116.0375) -> (68.9125, 103.0375)
  arc A113 (68.4125, 102.5375) -> (68.9125, 103.0375) centre (68.4125, 103.0375) ccw
  line L147 (68.4125, 102.5375) -> (55.4125, 102.5375)
  arc A114 (78.725, 26.8375) -> (79.225, 26.3375) centre (79.225, 26.8375) ccw
  line L148 (78.725, 26.8375) -> (78.725, 39.8375)
  arc A115 (79.225, 40.3375) -> (78.725, 39.8375) centre (79.225, 39.8375) ccw
  line L149 (79.225, 40.3375) -> (92.225, 40.3375)
  arc A116 (92.725, 39.8375) -> (92.225, 40.3375) centre (92.225, 39.8375) ccw
  line L150 (92.725, 39.8375) -> (92.725, 26.8375)
  arc A117 (92.225, 26.3375) -> (92.725, 26.8375) centre (92.225, 26.8375) ccw
  line L151 (92.225, 26.3375) -> (79.225, 26.3375)
  arc A118 (140.6375, 3.025) -> (141.1375, 2.525) centre (141.1375, 3.025) ccw
  line L152 (140.6375, 3.025) -> (140.6375, 16.025)
  arc A119 (141.1375, 16.525) -> (140.6375, 16.025) centre (141.1375, 16.025) ccw
  line L153 (141.1375, 16.525) -> (154.1375, 16.525)
  arc A120 (154.6375, 16.025) -> (154.1375, 16.525) centre (154.1375, 16.025) ccw
  line L154 (154.6375, 16.025) -> (154.6375, 3.025)
  arc A121 (154.1375, 2.525) -> (154.6375, 3.025) centre (154.1375, 3.025) ccw
  line L155 (154.1375, 2.525) -> (141.1375, 2.525)
  arc A122 (2.525, 3.025) -> (3.025, 2.525) centre (3.025, 3.025) ccw
  line L156 (2.525, 3.025) -> (2.525, 16.025)
  arc A123 (3.025, 16.525) -> (2.525, 16.025) centre (3.025, 16.025) ccw
  line L157 (3.025, 16.525) -> (16.025, 16.525)
  arc A124 (16.525, 16.025) -> (16.025, 16.525) centre (16.025, 16.025) ccw
  line L158 (16.525, 16.025) -> (16.525, 3.025)
  arc A125 (16.025, 2.525) -> (16.525, 3.025) centre (16.025, 3.025) ccw
  line L159 (16.025, 2.525) -> (3.025, 2.525)
  arc A126 (73.9625, 3.025) -> (74.4625, 2.525) centre (74.4625, 3.025) ccw
  line L160 (73.9625, 3.025) -> (73.9625, 16.025)
  arc A127 (74.4625, 16.525) -> (73.9625, 16.025) centre (74.4625, 16.025) ccw
  line L161 (74.4625, 16.525) -> (87.4625, 16.525)
  arc A128 (87.9625, 16.025) -> (87.4625, 16.525) centre (87.4625, 16.025) ccw
  line L162 (87.9625, 16.025) -> (87.9625, 3.025)
  arc A129 (87.4625, 2.525) -> (87.9625, 3.025) centre (87.4625, 3.025) ccw
  line L163 (87.4625, 2.525) -> (74.4625, 2.525)
  arc A130 (93.0125, 3.025) -> (93.5125, 2.525) centre (93.5125, 3.025) ccw
  line L164 (93.0125, 3.025) -> (93.0125, 16.025)
  arc A131 (93.5125, 16.525) -> (93.0125, 16.025) centre (93.5125, 16.025) ccw
  line L165 (93.5125, 16.525) -> (106.5125, 16.525)
  arc A132 (107.0125, 16.025) -> (106.5125, 16.525) centre (106.5125, 16.025) ccw
  line L166 (107.0125, 16.025) -> (107.0125, 3.025)
  arc A133 (106.5125, 2.525) -> (107.0125, 3.025) centre (106.5125, 3.025) ccw
  line L167 (106.5125, 2.525) -> (93.5125, 2.525)
  arc A134 (145.4, 45.8875) -> (145.9, 45.3875) centre (145.9, 45.8875) ccw
  line L168 (145.4, 45.8875) -> (145.4, 58.8875)
  arc A135 (145.9, 59.3875) -> (145.4, 58.8875) centre (145.9, 58.8875) ccw
  line L169 (145.9, 59.3875) -> (158.9, 59.3875)
  arc A136 (159.4, 58.8875) -> (158.9, 59.3875) centre (158.9, 58.8875) ccw
  line L170 (159.4, 58.8875) -> (159.4, 45.8875)
  arc A137 (158.9, 45.3875) -> (159.4, 45.8875) centre (158.9, 45.8875) ccw
  line L171 (158.9, 45.3875) -> (145.9, 45.3875)
  arc A138 (54.9125, 3.025) -> (55.4125, 2.525) centre (55.4125, 3.025) ccw
  line L172 (54.9125, 3.025) -> (54.9125, 16.025)
  arc A139 (55.4125, 16.525) -> (54.9125, 16.025) centre (55.4125, 16.025) ccw
  line L173 (55.4125, 16.525) -> (68.4125, 16.525)
  arc A140 (68.9125, 16.025) -> (68.4125, 16.525) centre (68.4125, 16.025) ccw
  line L174 (68.9125, 16.025) -> (68.9125, 3.025)
  arc A141 (68.4125, 2.525) -> (68.9125, 3.025) centre (68.4125, 3.025) ccw
  line L175 (68.4125, 2.525) -> (55.4125, 2.525)
  arc A142 (107.3, 45.8875) -> (107.8, 45.3875) centre (107.8, 45.8875) ccw
  line L176 (107.3, 45.8875) -> (107.3, 58.8875)
  arc A143 (107.8, 59.3875) -> (107.3, 58.8875) centre (107.8, 58.8875) ccw
  line L177 (107.8, 59.3875) -> (120.8, 59.3875)
  arc A144 (121.3, 58.8875) -> (120.8, 59.3875) centre (120.8, 58.8875) ccw
  line L178 (121.3, 58.8875) -> (121.3, 45.8875)
  arc A145 (120.8, 45.3875) -> (121.3, 45.8875) centre (120.8, 45.8875) ccw
  line L179 (120.8, 45.3875) -> (107.8, 45.3875)
  arc A146 (116.825, 26.8375) -> (117.325, 26.3375) centre (117.325, 26.8375) ccw
  line L180 (116.825, 26.8375) -> (116.825, 39.8375)
  arc A147 (117.325, 40.3375) -> (116.825, 39.8375) centre (117.325, 39.8375) ccw
  line L181 (117.325, 40.3375) -> (130.325, 40.3375)
  arc A148 (130.825, 39.8375) -> (130.325, 40.3375) centre (130.325, 39.8375) ccw
  line L182 (130.825, 39.8375) -> (130.825, 26.8375)
  arc A149 (130.325, 26.3375) -> (130.825, 26.8375) centre (130.325, 26.8375) ccw
  line L183 (130.325, 26.3375) -> (117.325, 26.3375)
  arc A150 (126.35, 45.8875) -> (126.85, 45.3875) centre (126.85, 45.8875) ccw
  line L184 (126.35, 45.8875) -> (126.35, 58.8875)
  arc A151 (126.85, 59.3875) -> (126.35, 58.8875) centre (126.85, 58.8875) ccw
  line L185 (126.85, 59.3875) -> (139.85, 59.3875)
  arc A152 (140.35, 58.8875) -> (139.85, 59.3875) centre (139.85, 58.8875) ccw
  line L186 (140.35, 58.8875) -> (140.35, 45.8875)
  arc A153 (139.85, 45.3875) -> (140.35, 45.8875) centre (139.85, 45.8875) ccw
  line L187 (139.85, 45.3875) -> (126.85, 45.3875)
  arc A154 (54.9125, 64.9375) -> (55.4125, 64.4375) centre (55.4125, 64.9375) ccw
  line L188 (54.9125, 64.9375) -> (54.9125, 77.9375)
  arc A155 (55.4125, 78.4375) -> (54.9125, 77.9375) centre (55.4125, 77.9375) ccw
  line L189 (55.4125, 78.4375) -> (68.4125, 78.4375)
  arc A156 (68.9125, 77.9375) -> (68.4125, 78.4375) centre (68.4125, 77.9375) ccw
  line L190 (68.9125, 77.9375) -> (68.9125, 64.9375)
  arc A157 (68.4125, 64.4375) -> (68.9125, 64.9375) centre (68.4125, 64.9375) ccw
  line L191 (68.4125, 64.4375) -> (55.4125, 64.4375)
  arc A158 (73.9625, 64.9375) -> (74.4625, 64.4375) centre (74.4625, 64.9375) ccw
  line L192 (73.9625, 64.9375) -> (73.9625, 77.9375)
  arc A159 (74.4625, 78.4375) -> (73.9625, 77.9375) centre (74.4625, 77.9375) ccw
  line L193 (74.4625, 78.4375) -> (87.4625, 78.4375)
  arc A160 (87.9625, 77.9375) -> (87.4625, 78.4375) centre (87.4625, 77.9375) ccw
  line L194 (87.9625, 77.9375) -> (87.9625, 64.9375)
  arc A161 (87.4625, 64.4375) -> (87.9625, 64.9375) centre (87.4625, 64.9375) ccw
  line L195 (87.4625, 64.4375) -> (74.4625, 64.4375)
  arc A162 (35.8625, 3.025) -> (36.3625, 2.525) centre (36.3625, 3.025) ccw
  line L196 (35.8625, 3.025) -> (35.8625, 16.025)
  arc A163 (36.3625, 16.525) -> (35.8625, 16.025) centre (36.3625, 16.025) ccw
  line L197 (36.3625, 16.525) -> (49.3625, 16.525)
  arc A164 (49.8625, 16.025) -> (49.3625, 16.525) centre (49.3625, 16.025) ccw
  line L198 (49.8625, 16.025) -> (49.8625, 3.025)
  arc A165 (49.3625, 2.525) -> (49.8625, 3.025) centre (49.3625, 3.025) ccw
  line L199 (49.3625, 2.525) -> (36.3625, 2.525)
  arc A166 (135.875, 26.8375) -> (136.375, 26.3375) centre (136.375, 26.8375) ccw
  line L200 (135.875, 26.8375) -> (135.875, 39.8375)
  arc A167 (136.375, 40.3375) -> (135.875, 39.8375) centre (136.375, 39.8375) ccw
  line L201 (136.375, 40.3375) -> (149.375, 40.3375)
  arc A168 (149.875, 39.8375) -> (149.375, 40.3375) centre (149.375, 39.8375) ccw
  line L202 (149.875, 39.8375) -> (149.875, 26.8375)
  arc A169 (149.375, 26.3375) -> (149.875, 26.8375) centre (149.375, 26.8375) ccw
  line L203 (149.375, 26.3375) -> (136.375, 26.3375)
  arc A170 (7.2875, 45.8875) -> (7.7875, 45.3875) centre (7.7875, 45.8875) ccw
  line L204 (7.2875, 45.8875) -> (7.2875, 58.8875)
  arc A171 (7.7875, 59.3875) -> (7.2875, 58.8875) centre (7.7875, 58.8875) ccw
  line L205 (7.7875, 59.3875) -> (20.7875, 59.3875)
  arc A172 (21.2875, 58.8875) -> (20.7875, 59.3875) centre (20.7875, 58.8875) ccw
  line L206 (21.2875, 58.8875) -> (21.2875, 45.8875)
  arc A173 (20.7875, 45.3875) -> (21.2875, 45.8875) centre (20.7875, 45.8875) ccw
  line L207 (20.7875, 45.3875) -> (7.7875, 45.3875)
  arc A174 (93.0125, 64.9375) -> (93.5125, 64.4375) centre (93.5125, 64.9375) ccw
  line L208 (93.0125, 64.9375) -> (93.0125, 77.9375)
  arc A175 (93.5125, 78.4375) -> (93.0125, 77.9375) centre (93.5125, 77.9375) ccw